Autodesk Inventor part; units mm, degrees
(part 2 of 2)
  spline S102 degree 2 poles (53.6176, 34.0216) (53.6802, 34.0216) (53.7876, 33.95) (53.8681, 33.7711) (53.9038, 33.476) (53.9038, 33.2614) knots 0 0 0 1 2 3 4 4 4
  spline S103 degree 2 poles (53.9038, 33.2614) (53.9038, 33.0378) (53.8681, 32.7426) (53.7876, 32.5548) (53.6802, 32.4743) (53.6176, 32.4743) knots 0 0 0 1 2 3 4 4 4
  line L129 (53.6176, 32.4743) -> (50.702, 32.4743)
  line L130 (50.702, 32.4743) -> (50.702, 28.9416)
  spline S104 degree 2 poles (50.702, 28.9416) (50.702, 28.8611) (50.6126, 28.7448) (50.389, 28.6643) (50.0223, 28.6196) (49.7361, 28.6196) knots 0 0 0 1 2 3 4 4 4
  spline S105 degree 2 poles (49.7361, 28.6196) (49.4588, 28.6196) (49.0832, 28.6643) (48.8686, 28.7448) (48.7702, 28.8611) (48.7702, 28.9416) knots 0 0 0 1 2 3 4 4 4
  line L131 (48.7702, 28.9416) -> (48.7702, 37.5364)
  spline S106 degree 2 poles (48.7702, 37.5364) (48.7702, 37.8584) (49.1011, 38.1446) (49.3426, 38.1446) knots 0 0 0 1 2 2 2
  line L132 (49.3426, 38.1446) -> (53.8055, 38.1446)
  spline S107 degree 2 poles (53.8055, 38.1446) (53.8681, 38.1446) (53.9754, 38.0641) (54.0559, 37.8852) (54.0917, 37.5722) (54.0917, 37.3576) knots 0 0 0 1 2 3 4 4 4
  spline S108 degree 2 poles (80.0212, 29.0356) (80.0212, 28.9641) (79.9228, 28.8478) (79.7081, 28.7763) (79.3414, 28.7316) (79.0642, 28.7316) knots 0 0 0 1 2 3 4 4 4
  spline S109 degree 2 poles (79.0642, 28.7316) (78.778, 28.7316) (78.4023, 28.7763) (78.1966, 28.8478) (78.0983, 28.9641) (78.0983, 29.0356) knots 0 0 0 1 2 3 4 4 4
  line L133 (78.0983, 29.0356) -> (78.0983, 32.8725)
  line L134 (78.0983, 32.8725) -> (74.5387, 32.8725)
  line L135 (74.5387, 32.8725) -> (74.5387, 29.0356)
  spline S110 degree 2 poles (74.5387, 29.0356) (74.5387, 28.9641) (74.4493, 28.8478) (74.2346, 28.7763) (73.8679, 28.7316) (73.5817, 28.7316) knots 0 0 0 1 2 3 4 4 4
  spline S111 degree 2 poles (73.5817, 28.7316) (73.3045, 28.7316) (72.9288, 28.7763) (72.7142, 28.8478) (72.6158, 28.9641) (72.6158, 29.0356) knots 0 0 0 1 2 3 4 4 4
  line L136 (72.6158, 29.0356) -> (72.6158, 37.9972)
  spline S112 degree 2 poles (72.6158, 37.9972) (72.6158, 38.0687) (72.7142, 38.185) (72.9288, 38.2566) (73.3045, 38.3013) (73.5817, 38.3013) knots 0 0 0 1 2 3 4 4 4
  spline S113 degree 2 poles (73.5817, 38.3013) (73.8679, 38.3013) (74.2346, 38.2566) (74.4493, 38.185) (74.5387, 38.0687) (74.5387, 37.9972) knots 0 0 0 1 2 3 4 4 4
  line L137 (74.5387, 37.9972) -> (74.5387, 34.5181)
  line L138 (74.5387, 34.5181) -> (78.0983, 34.5181)
  line L139 (78.0983, 34.5181) -> (78.0983, 37.9972)
  spline S114 degree 2 poles (78.0983, 37.9972) (78.0983, 38.0687) (78.1966, 38.185) (78.4023, 38.2566) (78.778, 38.3013) (79.0642, 38.3013) knots 0 0 0 1 2 3 4 4 4
  spline S115 degree 2 poles (79.0642, 38.3013) (79.3414, 38.3013) (79.7081, 38.2566) (79.9228, 38.185) (80.0212, 38.0687) (80.0212, 37.9972) knots 0 0 0 1 2 3 4 4 4
  line L140 (80.0212, 37.9972) -> (80.0212, 29.0356)
  spline S116 degree 2 poles (98.3727, 31.8136) (98.3727, 31.0623) (97.8182, 29.9354) (96.8612, 29.1841) (95.5912, 28.7996) (94.8668, 28.7996) knots 0 0 0 1 2 3 4 4 4
  spline S117 degree 2 poles (94.8668, 28.7996) (94.3749, 28.7996) (93.5342, 28.9605) (92.8903, 29.1931) (92.452, 29.4435) (92.2642, 29.6313) (92.1837, 29.9891) (92.1837, 30.3289) knots 0 0 0 1 2 3 4 5 6 6 6
  spline S118 degree 2 poles (92.1837, 30.3289) (92.1837, 30.5525) (92.2105, 30.8655) (92.2821, 31.0534) (92.3894, 31.1339) (92.461, 31.1339) knots 0 0 0 1 2 3 4 4 4
  spline S119 degree 2 poles (92.461, 31.1339) (92.5683, 31.1339) (92.935, 30.8924) (93.5253, 30.5972) (94.3391, 30.3558) (94.8668, 30.3558) knots 0 0 0 1 2 3 4 4 4
  spline S120 degree 2 poles (94.8668, 30.3558) (95.2246, 30.3558) (95.7791, 30.5257) (96.1636, 30.8298) (96.3693, 31.2859) (96.3693, 31.5631) knots 0 0 0 1 2 3 4 4 4
  spline S121 degree 2 poles (96.3693, 31.5631) (96.3693, 31.8851) (96.0205, 32.3502) (95.4571, 32.7079) (94.7416, 33.021) (93.9724, 33.3698) (93.2569, 33.817) (92.6935, 34.443) (92.3447, 35.2927) (92.3447, 35.8829) knots 0 0 0 1 2 3 4 5 6 7 8 8 8
  spline S122 degree 2 poles (92.3447, 35.8829) (92.3447, 36.5716) (92.8545, 37.6001) (93.7041, 38.2798) (94.8757, 38.6197) (95.5286, 38.6197) knots 0 0 0 1 2 3 4 4 4
  spline S123 degree 2 poles (95.5286, 38.6197) (95.8596, 38.6197) (96.5393, 38.5213) (97.1206, 38.3424) (97.5767, 38.1189) (97.7288, 37.9758) (97.7735, 37.8774) (97.8093, 37.7074) (97.8272, 37.4481) (97.8272, 37.2603) knots 0 0 0 1 2 3 4 5 6 7 8 8 8
  spline S124 degree 2 poles (97.8272, 37.2603) (97.8272, 37.0456) (97.8093, 36.7505) (97.7556, 36.5627) (97.6572, 36.4732) (97.5767, 36.4732) knots 0 0 0 1 2 3 4 4 4
  spline S125 degree 2 poles (97.5767, 36.4732) (97.4962, 36.4732) (97.1474, 36.6789) (96.6287, 36.9204) (95.9579, 37.1172) (95.5555, 37.1172) knots 0 0 0 1 2 3 4 4 4
  spline S126 degree 2 poles (95.5555, 37.1172) (95.2424, 37.1172) (94.7684, 36.9651) (94.4554, 36.6879) (94.3034, 36.3122) (94.3034, 36.0976) knots 0 0 0 1 2 3 4 4 4
  spline S127 degree 2 poles (94.3034, 36.0976) (94.3034, 35.7846) (94.6432, 35.3195) (95.2246, 34.9617) (95.9579, 34.6487) (96.7181, 34.2999) (97.4515, 33.8527) (98.0239, 33.2267) (98.3727, 32.386) (98.3727, 31.8136) knots 0 0 0 1 2 3 4 5 6 7 8 8 8
  spline S128 degree 2 poles (117.6606, 37.4346) (117.6606, 37.211) (117.6249, 36.9069) (117.5444, 36.737) (117.437, 36.6476) (117.3744, 36.6476) knots 0 0 0 1 2 3 4 4 4
  line L141 (117.3744, 36.6476) -> (114.271, 36.6476)
  line L142 (114.271, 36.6476) -> (114.271, 34.0986)
  line L143 (114.271, 34.0986) -> (117.1866, 34.0986)
  spline S129 degree 2 poles (117.1866, 34.0986) (117.2492, 34.0986) (117.3566, 34.0271) (117.437, 33.8482) (117.4728, 33.5531) (117.4728, 33.3384) knots 0 0 0 1 2 3 4 4 4
  spline S130 degree 2 poles (117.4728, 33.3384) (117.4728, 33.1148) (117.437, 32.8197) (117.3566, 32.6319) (117.2492, 32.5514) (117.1866, 32.5514) knots 0 0 0 1 2 3 4 4 4
  line L144 (117.1866, 32.5514) -> (114.271, 32.5514)
  line L145 (114.271, 32.5514) -> (114.271, 29.0186)
  spline S131 degree 2 poles (114.271, 29.0186) (114.271, 28.9381) (114.1816, 28.8219) (113.958, 28.7414) (113.5913, 28.6967) (113.3051, 28.6967) knots 0 0 0 1 2 3 4 4 4
  spline S132 degree 2 poles (113.3051, 28.6967) (113.0278, 28.6967) (112.6522, 28.7414) (112.4375, 28.8219) (112.3392, 28.9381) (112.3392, 29.0186) knots 0 0 0 1 2 3 4 4 4
  line L146 (112.3392, 29.0186) -> (112.3392, 37.6135)
  spline S133 degree 2 poles (112.3392, 37.6135) (112.3392, 37.9355) (112.6701, 38.2217) (112.9116, 38.2217) knots 0 0 0 1 2 2 2
  line L147 (112.9116, 38.2217) -> (117.3744, 38.2217)
  spline S134 degree 2 poles (117.3744, 38.2217) (117.437, 38.2217) (117.5444, 38.1412) (117.6249, 37.9623) (117.6606, 37.6493) (117.6606, 37.4346) knots 0 0 0 1 2 3 4 4 4
  spline S135 degree 2 poles (143.5362, 28.9509) (143.5362, 28.8793) (143.4378, 28.7631) (143.2232, 28.6915) (142.8565, 28.6468) (142.5792, 28.6468) knots 0 0 0 1 2 3 4 4 4
  spline S136 degree 2 poles (142.5792, 28.6468) (142.293, 28.6468) (141.9174, 28.6915) (141.7117, 28.7631) (141.6133, 28.8793) (141.6133, 28.9509) knots 0 0 0 1 2 3 4 4 4
  line L148 (141.6133, 28.9509) -> (141.6133, 32.7877)
  line L149 (141.6133, 32.7877) -> (138.0537, 32.7877)
  line L150 (138.0537, 32.7877) -> (138.0537, 28.9509)
  spline S137 degree 2 poles (138.0537, 28.9509) (138.0537, 28.8793) (137.9643, 28.7631) (137.7496, 28.6915) (137.3829, 28.6468) (137.0968, 28.6468) knots 0 0 0 1 2 3 4 4 4
  spline S138 degree 2 poles (137.0968, 28.6468) (136.8195, 28.6468) (136.4439, 28.6915) (136.2292, 28.7631) (136.1308, 28.8793) (136.1308, 28.9509) knots 0 0 0 1 2 3 4 4 4
  line L151 (136.1308, 28.9509) -> (136.1308, 37.9124)
  spline S139 degree 2 poles (136.1308, 37.9124) (136.1308, 37.984) (136.2292, 38.1002) (136.4439, 38.1718) (136.8195, 38.2165) (137.0968, 38.2165) knots 0 0 0 1 2 3 4 4 4
  spline S140 degree 2 poles (137.0968, 38.2165) (137.3829, 38.2165) (137.7496, 38.1718) (137.9643, 38.1002) (138.0537, 37.984) (138.0537, 37.9124) knots 0 0 0 1 2 3 4 4 4
  line L152 (138.0537, 37.9124) -> (138.0537, 34.4333)
  line L153 (138.0537, 34.4333) -> (141.6133, 34.4333)
  line L154 (141.6133, 34.4333) -> (141.6133, 37.9124)
  spline S141 degree 2 poles (141.6133, 37.9124) (141.6133, 37.984) (141.7117, 38.1002) (141.9174, 38.1718) (142.293, 38.2165) (142.5792, 38.2165) knots 0 0 0 1 2 3 4 4 4
  spline S142 degree 2 poles (142.5792, 38.2165) (142.8565, 38.2165) (143.2232, 38.1718) (143.4378, 38.1002) (143.5362, 37.984) (143.5362, 37.9124) knots 0 0 0 1 2 3 4 4 4
  line L155 (143.5362, 37.9124) -> (143.5362, 28.9509)
  spline S143 degree 2 poles (161.8878, 31.7288) (161.8878, 30.9775) (161.3332, 29.8506) (160.3763, 29.0994) (159.1063, 28.7148) (158.3818, 28.7148) knots 0 0 0 1 2 3 4 4 4
  spline S144 degree 2 poles (158.3818, 28.7148) (157.8899, 28.7148) (157.0492, 28.8758) (156.4053, 29.1083) (155.9671, 29.3587) (155.7792, 29.5466) (155.6987, 29.9043) (155.6987, 30.2442) knots 0 0 0 1 2 3 4 5 6 6 6
  spline S145 degree 2 poles (155.6987, 30.2442) (155.6987, 30.4678) (155.7256, 30.7808) (155.7971, 30.9686) (155.9044, 31.0491) (155.976, 31.0491) knots 0 0 0 1 2 3 4 4 4
  spline S146 degree 2 poles (155.976, 31.0491) (156.0833, 31.0491) (156.45, 30.8076) (157.0403, 30.5125) (157.8542, 30.271) (158.3818, 30.271) knots 0 0 0 1 2 3 4 4 4
  spline S147 degree 2 poles (158.3818, 30.271) (158.7396, 30.271) (159.2941, 30.4409) (159.6787, 30.745) (159.8844, 31.2011) (159.8844, 31.4784) knots 0 0 0 1 2 3 4 4 4
  spline S148 degree 2 poles (159.8844, 31.4784) (159.8844, 31.8004) (159.5356, 32.2654) (158.9721, 32.6232) (158.2566, 32.9362) (157.4875, 33.285) (156.772, 33.7322) (156.2085, 34.3582) (155.8597, 35.2079) (155.8597, 35.7982) knots 0 0 0 1 2 3 4 5 6 7 8 8 8
  spline S149 degree 2 poles (155.8597, 35.7982) (155.8597, 36.4868) (156.3695, 37.5154) (157.2192, 38.1951) (158.3908, 38.5349) (159.0437, 38.5349) knots 0 0 0 1 2 3 4 4 4
  spline S150 degree 2 poles (159.0437, 38.5349) (159.3746, 38.5349) (160.0543, 38.4366) (160.6356, 38.2577) (161.0918, 38.0341) (161.2438, 37.891) (161.2885, 37.7926) (161.3243, 37.6227) (161.3422, 37.3633) (161.3422, 37.1755) knots 0 0 0 1 2 3 4 5 6 7 8 8 8
  spline S151 degree 2 poles (161.3422, 37.1755) (161.3422, 36.9609) (161.3243, 36.6657) (161.2706, 36.4779) (161.1723, 36.3885) (161.0918, 36.3885) knots 0 0 0 1 2 3 4 4 4
  spline S152 degree 2 poles (161.0918, 36.3885) (161.0113, 36.3885) (160.6625, 36.5942) (160.1437, 36.8356) (159.473, 37.0324) (159.0705, 37.0324) knots 0 0 0 1 2 3 4 4 4
  spline S153 degree 2 poles (159.0705, 37.0324) (158.7575, 37.0324) (158.2835, 36.8804) (157.9704, 36.6031) (157.8184, 36.2275) (157.8184, 36.0128) knots 0 0 0 1 2 3 4 4 4
  spline S154 degree 2 poles (157.8184, 36.0128) (157.8184, 35.6998) (158.1582, 35.2347) (158.7396, 34.877) (159.473, 34.564) (160.2332, 34.2151) (160.9666, 33.768) (161.539, 33.1419) (161.8878, 32.3012) (161.8878, 31.7288) knots 0 0 0 1 2 3 4 5 6 7 8 8 8
  spline S155 degree 2 poles (181.1757, 37.3499) (181.1757, 37.1263) (181.1399, 36.8222) (181.0594, 36.6523) (180.9521, 36.5628) (180.8895, 36.5628) knots 0 0 0 1 2 3 4 4 4
  line L156 (180.8895, 36.5628) -> (177.786, 36.5628)
  line L157 (177.786, 36.5628) -> (177.786, 34.0139)
  line L158 (177.786, 34.0139) -> (180.7017, 34.0139)
  spline S156 degree 2 poles (180.7017, 34.0139) (180.7643, 34.0139) (180.8716, 33.9423) (180.9521, 33.7635) (180.9879, 33.4683) (180.9879, 33.2537) knots 0 0 0 1 2 3 4 4 4
  spline S157 degree 2 poles (180.9879, 33.2537) (180.9879, 33.0301) (180.9521, 32.7349) (180.8716, 32.5471) (180.7643, 32.4666) (180.7017, 32.4666) knots 0 0 0 1 2 3 4 4 4
  line L159 (180.7017, 32.4666) -> (177.786, 32.4666)
  line L160 (177.786, 32.4666) -> (177.786, 28.9339)
  spline S158 degree 2 poles (177.786, 28.9339) (177.786, 28.8534) (177.6966, 28.7371) (177.473, 28.6566) (177.1063, 28.6119) (176.8201, 28.6119) knots 0 0 0 1 2 3 4 4 4
  spline S159 degree 2 poles (176.8201, 28.6119) (176.5429, 28.6119) (176.1672, 28.6566) (175.9526, 28.7371) (175.8542, 28.8534) (175.8542, 28.9339) knots 0 0 0 1 2 3 4 4 4
  line L161 (175.8542, 28.9339) -> (175.8542, 37.5287)
  spline S160 degree 2 poles (175.8542, 37.5287) (175.8542, 37.8507) (176.1851, 38.1369) (176.4266, 38.1369) knots 0 0 0 1 2 2 2
  line L162 (176.4266, 38.1369) -> (180.8895, 38.1369)
  spline S161 degree 2 poles (180.8895, 38.1369) (180.9521, 38.1369) (181.0594, 38.0564) (181.1399, 37.8775) (181.1757, 37.5645) (181.1757, 37.3499) knots 0 0 0 1 2 3 4 4 4
  point P0 (0, 0)
  constraints: 36 other
emboss "Emboss2" sketch "Sketch6" operation cut depth 1.27 direction (0, 0, -1) contours S0 S1 L73 L74 L75 S2 S3 L76 S4 S5 L77 L78 L79 S6 S7 L80 | S8 S9 S10 S11 S12 S13 S14 S15 S16 S17 S18 S19 | S20 S21 L81 L82 L83 S22 S23 L84 S24 S25 L85 L86 L87 S26 S27 L88 | S28 L89 L90 L91 S29 S30 L92 L93 S31 S32 L94 S33 L95 S34 | S35 S36 S37 S38 S39 S40 S41 S42 S43 S44 S45 S46 | S47 L96 L97 L98 S48 S49 L99 L100 S50 S51 L101 S52 L102 S53 | S54 S55 L103 L104 L105 S56 S57 L106 S58 S59 L107 L108 L109 S60 S61 L110 | S62 S63 S64 S65 S66 S67 S68 S69 S70 S71 S72 S73 | S74 L111 L112 L113 S75 S76 L114 L115 S77 S78 L116 S79 L117 S80 | S81 S82 L118 L119 L120 S83 S84 L121 S85 S86 L122 L123 L124 S87 S88 L125 | S89 S90 S91 S92 S93 S94 S95 S96 S97 S98 S99 S100 | S101 L126 L127 L128 S102 S103 L129 L130 S104 S105 L131 S106 L132 S107 | S108 S109 L133 L134 L135 S110 S111 L136 S112 S113 L137 L138 L139 S114 S115 L140 | S116 S117 S118 S119 S120 S121 S122 S123 S124 S125 S126 S127 | S128 L141 L142 L143 S129 S130 L144 L145 S131 S132 L146 S133 L147 S134 | S135 S136 L148 L149 L150 S137 S138 L151 S139 S140 L152 L153 L154 S141 S142 L155 | S143 S144 S145 S146 S147 S148 S149 S150 S151 S152 S153 S154 | S155 L156 L157 L158 S156 S157 L159 L160 S158 S159 L161 S160 L162 S161
body "Solid1"
